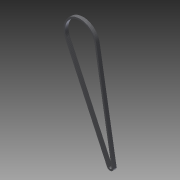
# Autodesk Inventor part: proxy chain 1
Saved by Autodesk Inventor 2011 SP1 (Build 150282100, 282)
## iProperties
Created: 2012-01-20
Part Number: proxy chain 1
Document SubType Name: Modeling
Designer: Christopher
Density: 1 g/cm^3
Author: Christopher
Autodesk Inventor part; units mm, degrees
ref_plane "YZ Plane" through (0, 0, 0) normal (1, 0, 0) x (0, 1, 0)
ref_plane "XZ Plane" through (0, 0, 0) normal (0, 1, 0) x (-1, 0, 0)
ref_plane "XY Plane" through (0, 0, 0) normal (0, 0, 1) x (1, 0, 0)
sketch "Sketch1" plane through (0, 0, 0) normal (0, 0, 1) x (1, 0, 0)
  line L0 (30.9216, 189.4198) -> (63.3973, -1.1372)
  line L1 (-28.8193, 170.8268) -> (51.3861, -2.6646)
  line L2 (27.7918, 188.8864) -> (60.1566, -1.0202)
  line L3 (54.2681, -1.3323) -> (-25.9374, 172.1591)
  arc A0 (54.2681, -1.3323) -> (60.1566, -1.0202) centre (57.15, 0) ccw
  arc A1 (51.3861, -2.6646) -> (63.3973, -1.1372) centre (57.15, 0) ccw
  arc A2 (27.7918, 188.8864) -> (-25.9374, 172.1591) centre (-0.1919, 184.1173) ccw
  arc A3 (30.9216, 189.4198) -> (-28.8193, 170.8268) centre (-0.1919, 184.1173) ccw
  point P0 (0, 0)
  point P1 (-0.3472, 183.9895)
  dimension "d4" = 3.175
  constraints: 8 end point, 8 point on circle, 4 centre point, 2 coincident, 2 tangent
  measures "d4" distance between parallel lines of L0 L2
extrude "Extrusion1" add sketch "Sketch1" against normal blind 6.35
body "Solid1"
